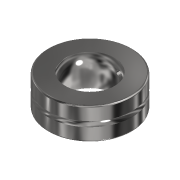
# Autodesk Inventor part: RBPB5h
Saved by Autodesk Inventor 2021 (Build 250183000, 183)
## iProperties
Part Number: RBPB5h
Material: Allgemein
Catalog Web Link: www.cadenas.de
Description: RBPB_holder-Spherical Bearings - Standard Type
Vendor: MISUMI
Document SubType Name: Modeling
Designer: partserver
Manufacturer: MISUMI
Mass: 0.675215 g
Surface Area: 7.69021 cm^2
Volume: 0.675215 cm^3
Density: 1 g/cm^3
Appearance: Stahl - poliert
Category: PARTsolutions
Company: MISUMI
PSOL_IDENT_0: {$CADENAS_DATA\23d-libs\misumi\metric\34_cylinders\rbpb_holder.prj},156 {VTYP=3D},{NB=RBPB5h},{LINA=
PSOL_IDENT_1: RBPB5},{NN=RBPB_holder},{DATE=04.06.2021 00:06:13},{GEOMDATE=18.05.2021 09:21:39},{VERSION=},{LINEID=
PSOL_IDENT_2: 10},{WBVAR=},{WBNUMERIC=}  {NB=RBPB5h},{LINA=RBPB5},{KT=DUMMY},{PN=RBPB5},{TYPE=RBPB},{MATH=1035 Ste
PSOL_IDENT_3: el},{MATSIR=51200 Bearing Steel},{STSIR=Hard Chrome Plating},{HARDSIR=58HRC~},{MATB=Special Copper A
PSOL_IDENT_4: lloy},{DD=5},{D=16},{B=6.00},{B1=8},{DD1=7.7},{H=1.0},{R=0.3},{BD=11.112},{A1=8},{A11=8},{A2=13},{A3=
PSOL_IDENT_5: 30},{SLC=7.84},{SLC1=7.84},{MASS=8.5},{RDC=0.035mm or Less},{ADC=0.1mm or Less},{HR=0.06}
NB: RBPB5h
NN: RBPB_holder
NT: Spherical Bearings - Standard Type
NBSYN: $PN.h
LINA: RBPB5
CATALOG: Misumi
MATSIR: 51200 Bearing Steel
DD: 5
D: 16
B: 6
B1: 8
DD1: 7.7
H: 1
R: 0.3
BD: 11.112
A11: 8
A2: 13
A3: 30
SLC1: 7.84
MASS: 8.5
ADC: 0.1mm or Less
HR: 0.06
SUPPLIER: MISUMI
ARTICLENO: RBPB5h
BOMINFO: RBPB5
CREATOR: CADENAS GmbH
Title: RBPB5
Author: Cadenas PARTsolutions
Comments: Spherical Bearings - Standard Type
Autodesk Inventor part; units mm, degrees
sketch "Sketch_3" plane through (0, 0, 0) normal (1, 0, 0) x (0, 1, 0)
  line L0 (0, -4) -> (0, 4)
  line L1 (0, 4) -> (3.8561, 4)
  arc A0 (3.8561, -4) -> (3.8561, 4) centre (0, 0) ccw
  line L2 (3.8561, -4) -> (0, -4)
  line L3 (0, -4) -> (0, 4)
  constraints: 8 end point, 2 point on circle, 1 centre point
sketch "Sketch_2" plane through (0, 0, 0) normal (1, 0, 0) x (0, 1, 0)
  line L0 (0, -3) -> (0, 3)
  line L1 (0, 3) -> (7.7, 3)
  arc A0 (8, 2.7) -> (7.7, 3) centre (7.7, 2.7) ccw
  line L2 (8, 2.7) -> (8, 0.5)
  arc A1 (8, 0.5) -> (8, -0.5) centre (10.0533, 0) ccw
  line L3 (8, -0.5) -> (8, -2.7)
  arc A2 (7.7, -3) -> (8, -2.7) centre (7.7, -2.7) ccw
  line L4 (7.7, -3) -> (0, -3)
  line L5 (0, -3) -> (0, 3)
  constraints: 12 end point, 6 point on circle, 3 centre point
revolve "Revolution1" add sketch "Sketch_2" angle 360 about axis through (0, 0, -3) along (0, 0, -1)
revolve "Revolution2" cut sketch "Sketch_3" angle 360 about axis through (0, 0, -4) along (0, 0, -1)
sketch "_____1" plane through (0, 0, 0) normal (1, 0, 0) x (0, 0, -1)
  line L0 (0, -32) -> (0, 32)
  line L1 (0, 9) -> (0.5, 9)
  line L2 (0.5, 9) -> (0.5, 0)
  line L3 (0.5, 0) -> (0, 0)
  line L4 (0, 0) -> (0, 9)
  constraints: 10 end point
revolve "Revolution3" cut sketch "_____1" angle 360 about axis through (0, -32, 0) along (0, -1, 0)
ref_plane "holder_XY" through (0, 0, 0) normal (0, 0, 1) x (1, 0, 0)
ref_plane "holder_YZ" through (0, 0, 0) normal (1, 0, 0) x (0, 1, 0)
ref_plane "holder_ZX" through (0, 0, 0) normal (0, 1, 0) x (0, 0, 1)
body "Solid1"
